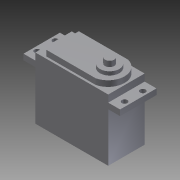
# Autodesk Inventor part: servo HS-7955GT
Saved by Autodesk Inventor 2012 (Build 160160000, 160)
## iProperties
Created: 2012-06-08
Part Number: servo HS-7955GT
Document SubType Name: Modeling
Designer: andi
Density: 1 g/cm^3
Material: Default
Author: andi
Autodesk Inventor part; units mm, degrees
ref_plane "YZ Plane" through (0, 0, 0) normal (1, 0, 0) x (0, 1, 0)
ref_plane "XZ Plane" through (0, 0, 0) normal (0, 1, 0) x (-1, 0, 0)
ref_plane "XY Plane" through (0, 0, 0) normal (0, 0, 1) x (1, 0, 0)
sketch "Sketch1" plane through (0, 0, 0) normal (0, 0, 1) x (1, 0, 0)
  line L0 (-19.557, 9.6136) -> (20.443, 9.6136)
  line L1 (20.443, 9.6136) -> (20.443, -10.3864)
  line L2 (20.443, -10.3864) -> (-19.557, -10.3864)
  line L3 (-19.557, -10.3864) -> (-19.557, 9.6136)
  point P0 (0, 0)
  dimension "d0" = 40
  dimension "d1" = 20
  constraints: 8 end point, 2 parallel, 1 horizontal, 1 perpendicular
  measures "d0" distance of L0.start L0.end
  measures "d1" distance of L2.end L0.start
extrude "Extrusion1" add sketch "Sketch1" along normal blind 37
sketch "Sketch2" plane through (0, 0, 37) normal (0, 0, 1) x (1, 0, 0)
  line L0 (20.443, 9.6136) -> (20.443, -10.3864) projected
  line L1 (-19.557, 9.6136) -> (20.443, 9.6136) projected
  line L2 (-19.557, -10.3864) -> (-19.557, 9.6136) projected
  line L3 (20.443, -10.3864) -> (-19.557, -10.3864) projected
  line L4 (-14.557, 8.4886) -> (12.443, 8.4886)
  line L5 (12.443, -9.2614) -> (-14.557, -9.2614)
  line L6 (-14.557, -9.2614) -> (-14.557, 8.4886)
  arc A0 (12.443, -9.2614) -> (12.443, 8.4886) centre (10.3169, -0.3864) ccw
  arc A1 (-14.557, 3.1386) -> (-14.557, -3.9114) centre (-11.6119, -0.3864) ccw
  point P0 (0, 0)
  dimension "d6" = 5
  dimension "d8" = 27
  dimension "d9" = 27
  dimension "d10" = 5.35
  dimension "d11" = 5.35
  constraints: 6 end point, 4 point on circle, 2 centre point, 2 point on line, 1 horizontal, 1 parallel
  measures "d6" distance between parallel lines of L2 L6
  measures "d8" distance from line of L4.end L6
  measures "d9" distance of L5.start L5.end
  measures "d10" distance from line of L4 A1.start
  measures "d11" distance of L5.end A1.end
extrude "Extrusion2" cut sketch "Sketch2" against normal blind 3.15
sketch "Sketch3" plane through (20.443, -10.3864, 0) normal (1, 0, 0) x (0, 0, -1)
  line L0 (-33.85, 20) -> (-33.85, 0) projected
  line L1 (0, 0) -> (-33.85, 0) projected
  line L2 (0, 20) -> (0, 0) projected
  line L3 (0, 20) -> (-33.85, 20) projected
  point P0 (0, 10.3864)
sketch "Sketch4" plane through (20.443, -10.3864, 0) normal (1, 0, 0) x (0, 0, -1)
  line L0 (-33.85, 20) -> (-33.85, 0) projected
  line L1 (0, 0) -> (-33.85, 0) projected
  line L2 (0, 20) -> (-33.85, 20) projected
  line L3 (-30, 20) -> (-26.85, 20)
  line L4 (-26.85, 20) -> (-26.85, 0)
  line L5 (-26.85, 0) -> (-30, 0)
  line L6 (-30, 0) -> (-30, 20)
  line L7 (-33.85, 0) -> (-33.85, 20) projected
  line L8 (0, 20) -> (-33.85, 20) projected
  line L9 (0, 0) -> (0, 20) projected
  line L10 (0, 0) -> (-33.85, 0) projected
  point P0 (0, 10.3864)
  dimension "d14" = 7
  dimension "d15" = 3.15
  constraints: 8 end point, 2 parallel, 2 point on line, 1 horizontal, 1 perpendicular
  measures "d14" distance between parallel lines of L4 L0
  measures "d15" distance between parallel lines of L4 L6
extrude "Extrusion3" add sketch "Sketch4" along normal blind 6.5 contours L2 L4 L1 L6
sketch "Sketch5" plane through (-19.557, -10.3864, 0) normal (-1, 0, 0) x (0, 0, 1)
  line L0 (33.85, 0) -> (33.85, 20) projected
  line L1 (0, 20) -> (33.85, 20) projected
  line L2 (0, 0) -> (33.85, 0) projected
  line L3 (26.85, 0) -> (30, 0)
  line L4 (30, 0) -> (30, 20)
  line L5 (30, 20) -> (26.85, 20)
  line L6 (26.85, 20) -> (26.85, 0)
  point P0 (0, 10.3864)
  dimension "d18" = 7
  dimension "d19" = 3.15
  constraints: 8 end point, 2 parallel, 2 point on line, 1 horizontal, 1 perpendicular
  measures "d18" distance between parallel lines of L0 L6
  measures "d19" distance between parallel lines of L4 L6
extrude "Extrusion4" add sketch "Sketch5" along normal blind 6.5 contours L2 L6 L1 L4
sketch "Sketch6" plane through (0, 0, 37) normal (0, 0, 1) x (1, 0, 0)
  circle A0 centre (11.193, -0.3864) radius 5.318
  line L0 (20.443, 9.6136) -> (20.443, -10.3864) projected
  circle A1 centre (11.193, -0.3864) radius 2.5
  point P0 (0, 0)
  dimension "d22" = 9.25
  dimension "d42" = 10.6361
  dimension "d75" = 5
  constraints: 2 centre point, 1 coincident
  measures "d22" distance from line of A0.centre L0
  measures "d42" diameter of A0
  measures "d75" diameter of A1
sketch "Sketch7" plane through (20.443, -10.3864, 30) normal (0, 0, 1) x (1, 0, 0)
  line L0 (6.5, 0) -> (6.5, 20) projected
  line L1 (0, 20) -> (6.5, 20) projected
  circle A0 centre (4, 5) radius 2.5
  circle A1 centre (4, 15) radius 2.5
  line L2 (0, 0) -> (0, 20) projected
  point P0 (-20.443, 10.3864)
  point P1 (5.6248, 3.1)
  point P2 (6.5, 3.3)
  point P3 (6.0702, 6.4015)
  point P4 (6.5, 6.3)
  point P5 (6, 13.5)
  point P6 (6.5, 13.7)
  point P7 (6, 16.5)
  point P8 (6.5, 16.7)
  dimension "d25" = 5
  dimension "d26" = 5
  dimension "d79" = 10
  dimension "d80" = 5
  dimension "d81" = 4
  dimension "d82" = 4
  constraints: 4 point on circle, 4 point on line, 2 centre point
  measures "d25" diameter of A0
  measures "d26" diameter of A1
  measures "d79" distance of A0.centre A1.centre
  measures "d80" distance from line of A1.centre L1
  measures "d81" distance from line of A1.centre L2
  measures "d82" distance from line of L2 A0.centre
sketch "Sketch8" plane through (-19.557, -10.3864, 30) normal (0, 0, 1) x (1, 0, 0)
  line L0 (-7.5004, 19.9995) -> (-7.5004, -0.0005)
  line L1 (-0.5, -0.0005) -> (-7.5004, -0.0005)
  line L2 (-0.4577, 19.9995) -> (-7.5004, 19.9995)
  circle A0 centre (-4, 14.9995) radius 2.5
  circle A1 centre (-4, 4.9995) radius 2.5
  line L3 (0, 20) -> (0, 0) projected
  point P0 (19.557, 10.3864)
  point P1 (-20.443, 10.3864)
  point P2 (-6, 16.4995)
  point P3 (-7.5004, 16.6995)
  point P4 (-6, 13.4995)
  point P5 (-7.5004, 13.6995)
  point P6 (-6, 6.4995)
  point P7 (-7.5004, 6.2995)
  point P8 (-6, 3.4995)
  point P9 (-7.5004, 3.2995)
  dimension "d35" = 5
  dimension "d36" = 5
  dimension "d37" = 5
  dimension "d38" = 5
  dimension "d83" = 10
  dimension "d84" = 4
  dimension "d85" = 4
  constraints: 6 end point, 4 point on circle, 4 point on line, 2 centre point
  measures "d35" distance from line of A0.centre L2
  measures "d36" distance from line of L1 A1.centre
  measures "d37" diameter of A0
  measures "d38" diameter of A1
  measures "d83" distance of A1.centre A0.centre
  measures "d84" distance from line of A0.centre L3
  measures "d85" distance from line of L3 A1.centre
extrude "Extrusion7" add sketch "Sketch6" along normal blind 2 contours A0 | A1
hole "Hole1" at (24.443, 4.6136, 30) at (24.443, -5.3864, 30) direction (0, 0, -1) diameter 3 end through all
hole "Hole2" at (-23.557, 4.6131, 30) at (-23.557, -5.3869, 30) direction (0, 0, -1) diameter 3 end through all
extrude "Extrusion14" add sketch "Sketch6" along normal blind 5 contours A1
body "Solid1"
